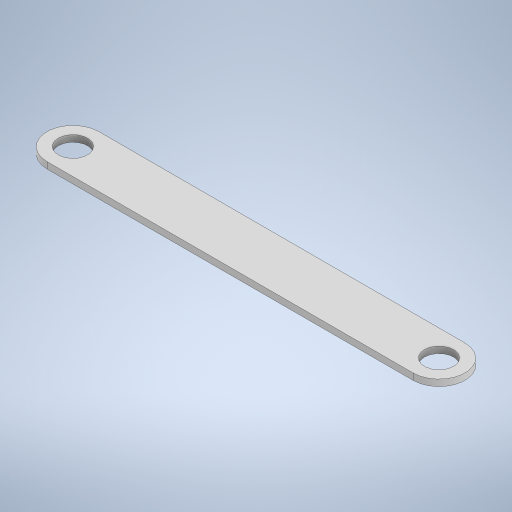
# Autodesk Inventor part: 4-bar intake (14.112) bar
Saved by Autodesk Inventor 2023 (Build 270158030, 158C)
## iProperties
Created: 2022-07-18
Part Number: 4-bar intake (14.112) bar
Material: Generic
Document SubType Name: Modeling
Designer: kt1040502
Density: 1 g/cm^3
Appearance: Default
Author: kt1040502
Autodesk Inventor part; units mm, degrees
ref_plane "YZ Plane" through (0, 0, 0) normal (1, 0, 0) x (0, 1, 0)
ref_plane "XZ Plane" through (0, 0, 0) normal (0, 1, 0) x (-1, 0, 0)
ref_plane "XY Plane" through (0, 0, 0) normal (0, 0, 1) x (1, 0, 0)
sketch "Sketch1" plane through (0, 0, 0) normal (0, 1, 0) x (-1, 0, 0)
  line L0 (0, 0) -> (-358.4448, 0)
  line L1 (0, 0) -> (-358.4448, 0) construction
  line L2 (0, 0) -> (-358.4448, 0) construction
  line L3 (0, 25.4) -> (-358.4448, 25.4)
  line L4 (-358.4448, -25.4) -> (0, -25.4)
  arc A0 (0, -25.4) -> (0, 25.4) centre (0, 0) ccw
  arc A1 (-358.4448, 25.4) -> (-358.4448, -25.4) centre (-358.4448, 0) ccw
  circle A2 centre (0, 0) radius 14.2875
  circle A3 centre (-358.4448, 0) radius 14.2875
  point P0 (-179.2224, 0)
  point P1 (-179.2224, 0)
  dimension "d0" = 358.4448
  dimension "d8" = 50.8
  dimension "d9" = 28.575
  dimension "d10" = 28.575
  constraints: 14 end point, 4 centre point, 4 point on circle, 4 tangent, 2 coincident, 2 equal length, 2 midpoint, 1 horizontal
  measures "d0" distance of L0.start L0.end
  measures "d8" diameter of A1
  measures "d9" diameter of A2
  measures "d10" diameter of A3
extrude "Extrusion1" add sketch "Sketch1" along normal blind 6.35
body "Solid1"
